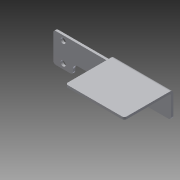
# Autodesk Inventor part: Circuit Breaker Mount
Saved by Autodesk Inventor 2013 (Build 170138000, 138)
## iProperties
Created: 2013-02-10
Part Number: Circuit Breaker Mount
Material: Aluminum 6061
Document SubType Name: Sheet Metal
Designer: Moses
Mass: 50.4305 g
Surface Area: 135.956 cm^2
Volume: 18.6091 cm^3
Density: 2.71 g/cm^3
Sheet Metal Rule: Default
Author: Moses
Autodesk Inventor part; units mm, degrees
ref_plane "YZ Plane" through (0, 0, 0) normal (1, 0, 0) x (0, 1, 0)
ref_plane "XZ Plane" through (0, 0, 0) normal (0, 1, 0) x (-1, 0, 0)
ref_plane "XY Plane" through (0, 0, 0) normal (0, 0, 1) x (1, 0, 0)
sketch "Sketch1" plane through (0, 0, 0) normal (0, 0, 1) x (1, 0, 0)
  line L0 (0, 0) -> (25.4, 0)
  line L1 (25.4, 0) -> (25.4, 38.1)
  line L2 (25.4, 38.1) -> (0, 38.1)
  line L3 (0, 38.1) -> (0, 0)
  line L4 (0, 19.05) -> (25.4, 19.05) construction
  line L5 (12.7, 31.75) -> (12.7, 6.35) construction
  circle A0 centre (12.7, 31.75) radius 3.302
  circle A1 centre (12.7, 6.35) radius 3.302
  line L6 (152.4, 38.1) -> (25.4, 38.1)
  line L7 (25.4, 12.7) -> (152.4, 12.7)
  line L8 (152.4, 12.7) -> (152.4, 38.1)
  line L9 (76.2, 38.1) -> (76.2, 41.275)
  line L10 (76.2, 41.275) -> (152.4, 41.275)
  line L11 (152.4, 41.275) -> (152.4, 38.1)
  point P0 (12.7, 19.05)
  dimension "d0" = 25.4
  dimension "d2" = 6.604
  dimension "d3" = 6.604
  dimension "d4" = 38.1
  dimension "d5" = 25.4
  dimension "d6" = 127
  dimension "d7" = 25.4
  dimension "d8" = 76.2
  dimension "d9" = 3.175
  measures "d0" distance of L5.start L5.end
  measures "d2" diameter of A0
  measures "d3" diameter of A1
  measures "d4" distance of L2.end L0.start
  measures "d5" distance of L1.end L2.end
  measures "d6" distance of L6.start L1.end
  measures "d7" distance of L7.end L6.start
  measures "d8" distance of L9.end L10.end
  measures "d9" distance of L9.start L9.end
extrude "Plate1" add sketch "Sketch1" along normal blind 3.048
sketch "Sketch2" plane through (76.2, 42.545, 4.318) normal (0, 1, 0) x (-1, 0, 0)
  line L0 (-76.2, 0) -> (0, 0)
  line L1 (0, 0) -> (0, 59.182)
  line L2 (0, 59.182) -> (-76.2, 59.182)
  line L3 (-76.2, 59.182) -> (-76.2, 0)
  constraints: 6 end point, 1 horizontal, 1 perpendicular, 1 vertical
edge flange "Flange1" height 63.5 angle 90 thickness 3.048 bend radius 1.27 thickness toward (0, 1, 0) relief straight relief width 3.048 relief depth 1.524 edges at (114.3, 41.275, 3.048) wall of the first edge with corners at (152.4, 42.545, 4.318) (76.2, 42.545, 4.318) (76.2, 42.545, 63.5) (152.4, 42.545, 63.5)
bend "Bend1"
corner "Corner1"
fillet "Corner Round1" radius 6.35 1 edges at (25.4, 12.7, 1.524)
fillet "Corner Round1" radius 3.175 7 edges at (0, 38.1, 1.524) (0, 0, 1.524) (25.4, 0, 1.524) (76.2, 44.069, 63.5) (152.4, 44.069, 63.5) (152.4, 12.7, 1.524) (76.2, 38.1, 1.524)
equation "\"d11\" = BendReliefWidth"
equation "\"d12\" = BendReliefDepth"
equation "\"d13\" = MinimumRemnant"
equation "\"d14\" = BendRadius"
equation "\"d18\" = CornerReliefSize"
equation "\"d19\" = GapSize"
equation "\"d20\" = JacobiRadiusSize"
equation "\"BendRadius\" = Thickness"
equation "\"BendReliefWidth\" = Thickness"
equation "\"BendReliefDepth\" = 0.5 * Thickness"
equation "\"CornerReliefSize\" = 4 * Thickness"
equation "\"MinimumRemnant\" = 2 * Thickness"
equation "\"TransitionRadius\" = BendRadius"
equation "\"JacobiRadiusSize\" = BendRadius"
equation "\"GapSize\" = Thickness"
equation "\"d10\" = BendRadius"
equation "\"Thickness\" = 3.048"
body "Solid1"
